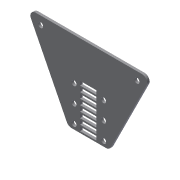
# Autodesk Inventor part: Belt plate base
Saved by Autodesk Inventor 2015 SP1 (Build 190203100, 203)
## iProperties
Created: 2015-01-18
Part Number: Belt plate base
Material: Generic
Document SubType Name: Sheet Metal
Designer: Owner
Density: 1 g/cm^3
Sheet Metal Rule: Default
Appearance: Default
Author: Owner
Autodesk Inventor part; units mm, degrees
ref_plane "YZ Plane" through (0, 0, 0) normal (1, 0, 0) x (0, 1, 0)
ref_plane "XZ Plane" through (0, 0, 0) normal (0, 1, 0) x (-1, 0, 0)
ref_plane "XY Plane" through (0, 0, 0) normal (0, 0, 1) x (1, 0, 0)
sketch "Sketch1" plane through (0, 0, 0) normal (0, 0, 1) x (1, 0, 0)
  line L0 (0, 0) -> (50.8, 0)
  line L1 (-50.8, 101.6) -> (101.6, 101.6)
  line L2 (50.8, 0) -> (101.6, 101.6)
  line L3 (-50.8, 101.6) -> (0, 0)
  line L4 (14.6239, 7) -> (34.6239, 7)
  line L5 (34.6239, 7) -> (34.6239, 2)
  line L6 (34.6239, 2) -> (14.6239, 2)
  line L7 (14.6239, 2) -> (14.6239, 7)
  line L8 (50.8, 0) -> (50.8, 62.4863)
  line L9 (14.6239, 14) -> (34.6239, 14)
  line L10 (34.6239, 14) -> (34.6239, 9)
  line L11 (34.6239, 9) -> (14.6239, 9)
  line L12 (14.6239, 9) -> (14.6239, 14)
  line L13 (14.6239, 21) -> (34.6239, 21)
  line L14 (34.6239, 21) -> (34.6239, 16)
  line L15 (34.6239, 16) -> (14.6239, 16)
  line L16 (14.6239, 16) -> (14.6239, 21)
  line L17 (14.6239, 28) -> (34.6239, 28)
  line L18 (34.6239, 28) -> (34.6239, 23)
  line L19 (34.6239, 23) -> (14.6239, 23)
  line L20 (14.6239, 23) -> (14.6239, 28)
  line L21 (14.6239, 35) -> (34.6239, 35)
  line L22 (34.6239, 35) -> (34.6239, 30)
  line L23 (34.6239, 30) -> (14.6239, 30)
  line L24 (14.6239, 30) -> (14.6239, 35)
  line L25 (14.6239, 42) -> (34.6239, 42)
  line L26 (34.6239, 42) -> (34.6239, 37)
  line L27 (34.6239, 37) -> (14.6239, 37)
  line L28 (14.6239, 37) -> (14.6239, 42)
  circle A0 centre (43.7057, 6.2222) radius 3.1623
  circle A1 centre (43.7057, 28) radius 3.1623
  circle A2 centre (43.7057, 49.7778) radius 3.1623
  line L29 (25.4, 0) -> (25.4, -15.6085)
  circle A3 centre (7.0943, 6.2222) radius 3.1623
  circle A4 centre (7.0943, 28) radius 3.1623
  circle A5 centre (7.0943, 49.7778) radius 3.1623
  line L30 (14.6239, 49) -> (34.6239, 49)
  line L31 (34.6239, 49) -> (34.6239, 44)
  line L32 (34.6239, 44) -> (14.6239, 44)
  line L33 (14.6239, 44) -> (14.6239, 49)
  line L34 (14.6239, 56) -> (34.6239, 56)
  line L35 (34.6239, 56) -> (34.6239, 51)
  line L36 (34.6239, 51) -> (14.6239, 51)
  line L37 (14.6239, 51) -> (14.6239, 56)
  circle A6 centre (-34.29, 91.44) radius 3.1623
  circle A7 centre (85.09, 91.44) radius 3.1623
  dimension "d0" = 50.8
  dimension "d1" = 152.4
  dimension "d2" = 101.6
  dimension "d5" = 50.8
  dimension "d6" = 20
  dimension "d7" = 5
  dimension "d8" = 2
  dimension "d11" = 7
  dimension "d16" = 6.3246
  dimension "d19" = 6.3246
  dimension "d21" = 6.3246
  dimension "d26" = 14
  dimension "d31" = 56
  dimension "d35" = 6.2222
  dimension "d36" = 6.2222
  dimension "d37" = 28
  dimension "d38" = 6.3246
  dimension "d39" = 6.3246
  dimension "d40" = 34.29
  dimension "d41" = 34.29
  dimension "d42" = 10.16
  dimension "d43" = 10.16
  dimension "d46" = 9.0818
  measures "d0" distance of L0.start L0.end
  measures "d1" distance of L1.start L1.end
  measures "d2" distance between parallel lines of L1 L0
  measures "d5" horizontal distance of L1.end L0.end
  measures "d6" distance of L5.end L6.end
  measures "d7" distance between parallel lines of L4 L6
  measures "d8" distance between parallel lines of L0 L6
  measures "d11" distance of L4.start L9.start
  measures "d16" diameter of A0
  measures "d19" diameter of A1
  measures "d21" diameter of A2
  measures "d26" distance of L23.end L32.end
  measures "d31" distance between parallel lines of L0 L34
  measures "d35" distance from line of L34 A2.centre
  measures "d36" distance from line of L0 A0.centre
  measures "d37" distance from line of L0 A1.centre
  measures "d38" diameter of A6
  measures "d39" diameter of A7
  measures "d40" horizontal distance of A7.centre L0.end
  measures "d41" horizontal distance of A6.centre L0.start
  measures "d42" vertical distance of A6.centre L1.start
  measures "d43" vertical distance of A7.centre L1.end
  measures "d46" distance from line of L35 A2.centre
extrude "Plate1" add sketch "Sketch1" along normal blind 3.048
fillet "Corner Round1" radius 6.35 4 edges at (101.6, 101.6, 1.524) (-50.8, 101.6, 1.524) (50.8, 0, 1.524) (0, 0, 1.524)
equation "\"d19\" = d16"
equation "\"d21\" = d19"
equation "\"d35\" = 0.111111 * d31"
equation "\"d36\" = d35"
equation "\"d37\" = 0.5 * d31"
equation "\"d41\" = d40"
equation "\"d43\" = d42"
equation "\"BendRadius\" = Thickness"
equation "\"BendReliefWidth\" = Thickness"
equation "\"BendReliefDepth\" = 0.5 * Thickness"
equation "\"CornerReliefSize\" = 4 * Thickness"
equation "\"MinimumRemnant\" = 2 * Thickness"
equation "\"TransitionRadius\" = BendRadius"
equation "\"JacobiRadiusSize\" = BendRadius"
equation "\"GapSize\" = Thickness"
equation "\"d44\" = BendRadius"
equation "\"Thickness\" = 3.048"
body "Solid1"
